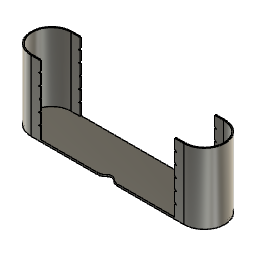
retractionTest (Autodesk Fusion 360 design; units mm, degrees)
Autodesk Fusion 360 part; units mm, degrees
sketch "Sketch1" plane through (0, 0, 0) normal (0, 0, 1) x (1, 0, 0)
  line L0 (0, 0) -> (-42.5, 0)
  line L1 (-42.5, 0) -> (-42.5, 18) construction
  line L2 (-42.5, 18) -> (0, 18)
  line L3 (0, 18) -> (0, 0)
  arc A0 (-33.5, 18) -> (-33.5, 0) centre (-33.5, 9) ccw
  line L4 (-33.5, 18) -> (-29.5, 18)
  line L5 (-33.5, 0) -> (-29.5, 0)
  line L6 (-33.5, 0.5) -> (-29.5, 0.5)
  arc A1 (-33.5, 17.5) -> (-33.5, 0.5) centre (-33.5, 9) ccw
  line L7 (-33.5, 17.5) -> (-29.5, 17.5)
  line L8 (-29.5, 18) -> (-29.5, 17.5)
  line L9 (-29.5, 0.5) -> (-29.5, 0)
  dimension "d6" = 42.5
  dimension "d7" = 18
  dimension "d8" = 4
  dimension "d9" = 4
  constraint horizontal L0
  constraint vertical L1
  constraint horizontal L2
  constraint vertical L3
  constraint coincident L0.start L3.end
  constraint tangent L2 A0
  constraint tangent L1 A0
  constraint tangent L0 A0
  constraint coincident L0 A0.end
  constraint coincident L2 A0.start
  constraint parallel L2 L4
  constraint parallel L0 L5
  constraint perpendicular L5 L9
  measures "d6" distance of L0.start L0.end
  measures "d7" distance of L0.start L2.end
  measures "d8" distance of A0.start L4.end
  measures "d9" distance of A0.end L5.end
extrude "Extrude1" add sketch "Sketch1" against normal blind 0.8
extrude "Extrude2" add sketch "Sketch1" along normal blind 30 contours L0 L2 A0 L4 L5 L6 A1 L7 L8 L9
sketch "Sketch2" plane through (0, 0, 0) normal (0, -1, 0) x (1, 0, 0)
  line L0 (-33.5, 30) -> (-33.5, -0.8)
  line L1 (-33.5, -0.8) -> (0, -0.8)
  line L2 (0, -0.8) -> (0, 0)
  line L3 (0, 0) -> (-29.5, 0)
  line L4 (-29.5, 0) -> (-29.5, 30)
  line L5 (-29.5, 30) -> (-33.5, 30)
  line L6 (-33.5, 0) -> (-29.5, 0)
  line L7 (-29.5, 5.7) -> (-30.2, 5)
  line L8 (-30.2, 5) -> (-29.5, 5)
  line L9 (-29.5, 5.7) -> (-29.5, 5)
  dimension "d31" = 0.7
  dimension "d32" = 45
  dimension "d33" = 5
  constraint coincident L4 L7.start
  constraint coincident L4 L8.end
  constraint perpendicular L4 L8
  measures "d31" distance of L7.start L8.end
  measures "d32" angle of L7 L8
  measures "d33" distance of L3.end L8.end
extrude "Extrude3" cut sketch "Sketch2" against normal through all contours L4 L7 L8 L9
pattern_linear "R-Pattern1" count 5 spacing 5 along (0, 0, 1) of "Extrude3"
mirror "Mirror1" about plane through (0, 0, 0) normal (1, 0, 0) of bodies 1 merged
sketch "Sketch3" plane through (0, 0, 0) normal (0, 0, 1) x (-1, 0, 0)
  arc A0 (-33.5, -0.5) -> (-33.5, -17.5) centre (-33.5, -9) ccw
  arc A1 (33.5, -17.5) -> (33.5, -0.5) centre (33.5, -9) ccw
  circle A2 centre (0, 0) radius 2
  line L0 (29.5, -0.5) -> (29.5, 0)
  line L1 (29.5, 0) -> (-29.5, 0)
  line L2 (-29.5, 0) -> (-29.5, -0.5)
  line L3 (-29.5, -0.5) -> (-33.5, -0.5)
  line L4 (-33.5, -17.5) -> (-29.5, -17.5)
  line L5 (-29.5, -17.5) -> (-29.5, -18)
  line L6 (-29.5, -18) -> (29.5, -18)
  line L7 (29.5, -18) -> (29.5, -17.5)
  line L8 (29.5, -17.5) -> (33.5, -17.5)
  line L9 (33.5, -0.5) -> (29.5, -0.5)
  dimension "d27" = 4
  constraint coincident A2.centre origin
  measures "d27" diameter of A2
extrude "Extrude4" cut sketch "Sketch3" against normal through all contours A2 L1 picked at (1.1554, -0.8465)
fillet "Fillet1" radius 4 2 edges at (-2, 0, -0.4) (2, 0, -0.4)
equation "baseThickness = 0.8 mm"
equation "baseLength = 85 mm"
equation "baseWidth = 18 mm"
equation "numSegments = 6"
equation "segmentHeight = 5 mm"
equation "d10 = -extrusionWidth"
equation "extrusionWidth = 0.5 mm"
equation "d12 = -baseThickness"
equation "d14 = numSegments * segmentHeight"
equation "layerHeight = 0.2 mm"
equation "d21 = numSegments - 1"
equation "d23 = segmentHeight"
equation "d31 = segmentNotchHeight"
equation "d33 = segmentHeight"
equation "segmentNotchHeight = 0.7 mm"
